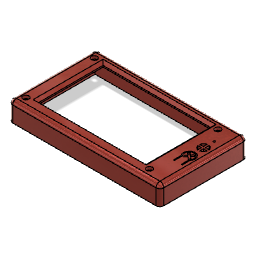
1-5i_Case_Front v4 (Autodesk Fusion 360 design; units mm, degrees)
Autodesk Fusion 360 part; units mm, degrees
sketch "Sketch1" plane through (0, 14.8501, 0) normal (0, 1, 0) x (-1, 0, 0)
  line L0 (118.407, 52.4604) -> (106.757, 52.4604)
  line L1 (106.757, 52.4604) -> (106.757, 50.3604)
  arc A0 (106.257, 49.8604) -> (106.757, 50.3604) centre (106.257, 50.3604) ccw
  line L2 (106.257, 49.8604) -> (103.757, 49.8604)
  line L3 (103.757, 49.8604) -> (103.757, 47.2604)
  arc A1 (103.257, 46.7604) -> (103.757, 47.2604) centre (103.257, 47.2604) ccw
  line L4 (103.257, 46.7604) -> (30.507, 46.7604)
  arc A2 (30.007, 47.2604) -> (30.507, 46.7604) centre (30.507, 47.2604) ccw
  line L5 (30.007, 47.2604) -> (30.007, 52.4604)
  line L6 (30.007, 52.4604) -> (-27.043, 52.4604)
  line L7 (-27.043, 52.4604) -> (-27.043, -23.3396)
  line L8 (-27.043, -23.3396) -> (118.407, -23.3396)
  line L9 (118.407, -23.3396) -> (118.407, 29.9604)
  line L10 (118.407, 29.9604) -> (116.257, 29.9604)
  arc A3 (115.757, 30.4604) -> (116.257, 29.9604) centre (116.257, 30.4604) ccw
  line L11 (115.757, 30.4604) -> (115.757, 43.4604)
  arc A4 (116.257, 43.9604) -> (115.757, 43.4604) centre (116.257, 43.4604) ccw
  line L12 (116.257, 43.9604) -> (118.407, 43.9604)
  line L13 (118.407, 43.9604) -> (118.407, 52.4604)
  circle A5 centre (115.807, 49.8604) radius 2.25
  circle A6 centre (115.807, -20.7396) radius 2.25
  circle A7 centre (-11.693, 49.8604) radius 2.25
  circle A8 centre (-11.693, -20.7396) radius 2.25
  circle A9 centre (115.807, 14.5604) radius 2.25
  circle A10 centre (115.807, -20.7396) radius 1.75
  circle A11 centre (115.807, 49.8604) radius 1.75
  circle A12 centre (-11.693, 49.8604) radius 1.75
  circle A13 centre (-11.693, -20.7396) radius 1.75
  circle A14 centre (-11.693, -20.7396) radius 3
  circle A15 centre (-11.693, 49.8604) radius 3
  circle A16 centre (115.807, 49.8604) radius 3
  circle A17 centre (115.807, -20.7396) radius 3
  dimension "d1" = 3.5
  dimension "d2" = 3.5
  dimension "d3" = 3.5
  dimension "d4" = 3.5
  dimension "d5" = 6
  dimension "d6" = 6
  dimension "d7" = 6
  dimension "d8" = 6
  constraint concentric A6 A10
  constraint concentric A5 A11
  constraint concentric A7 A12
  constraint concentric A8 A13
  constraint concentric A8 A14
  constraint concentric A7 A15
  constraint concentric A5 A16
  constraint concentric A6 A17
  measures "d1" diameter of A10
  measures "d2" diameter of A11
  measures "d3" diameter of A12
  measures "d4" diameter of A13
  measures "d5" diameter of A14
  measures "d6" diameter of A15
  measures "d7" diameter of A16
  measures "d8" diameter of A17
extrude "Extrude1" add sketch "Sketch1" along normal blind 4.3 contours L0 L13 A16 | L0 A16 | L13 A16 | L9 A17 | L8 L9 A17 | L8 A17 | L8 A14 | L8 A14 | L6 A15 | L6 A15 | A5 | A6 | A7 | A8 picked at (115.8631, 52.3416) picked at (115.751, -23.2209) makes body 1 at (-115.7322, 17.7168, 46.8613) makes body 2 at (8.7079, 17.7168, 50.1591) makes body 3 at (-116.6196, 16.2834, -23.6275) makes body 4 at (8.7079, 17.7168, -20.4409)
sketch "Sketch2" plane through (0, 19.1501, 0) normal (0, 1, 0) x (-1, 0, 0)
  circle A0 centre (115.807, -20.7396) radius 1.75
  circle A1 centre (115.807, -20.7396) radius 3
  line L0 (120.907, -26.5896) -> (-29.043, -26.5896)
  line L1 (-29.043, -26.5896) -> (-29.043, 56.4604)
  line L2 (-29.043, 56.4604) -> (120.907, 56.4604)
  line L3 (120.907, 56.4604) -> (120.907, -26.5896)
  line L4 (109.007, -23.0896) -> (-5.793, -23.0896)
  line L5 (-5.793, -23.0896) -> (-5.793, 45.4104)
  line L6 (-5.793, 45.4104) -> (109.007, 45.4104)
  line L7 (109.007, 45.4104) -> (109.007, -23.0896)
  line L8 (-27.043, -23.3396) -> (118.407, -23.3396)
  line L9 (108.757, -22.8396) -> (-5.543, -22.8396)
  line L10 (108.757, 45.1604) -> (108.757, -22.8396)
  line L11 (-5.543, 45.1604) -> (108.757, 45.1604)
  line L12 (-5.543, -22.8396) -> (-5.543, 45.1604)
  line L13 (110.507, -24.5896) -> (-8.293, -24.5896)
  line L14 (-27.043, 52.4604) -> (-27.043, -23.3396)
  circle A2 centre (115.807, 49.8604) radius 1.75
  circle A3 centre (-11.693, 49.8604) radius 1.75
  circle A4 centre (-11.693, -20.7396) radius 1.75
  circle A5 centre (-20.543, 2.9604) radius 5
  line L15 (-25.4419, 1.9604) -> (-15.644, 1.9604)
  line L16 (-15.644, 1.9604) -> (-15.644, 3.9604)
  line L17 (-15.644, 3.9604) -> (-25.4419, 3.9604)
  line L18 (-25.4419, 3.9604) -> (-25.4419, 1.9604)
  line L19 (-25.4419, 1.9604) -> (-15.644, 3.9604) construction
  line L20 (-15.644, 1.9604) -> (-25.4419, 3.9604) construction
  line L21 (-21.543, -1.9386) -> (-19.543, -1.9386)
  line L22 (-19.543, -1.9386) -> (-19.543, 7.8593)
  line L23 (-19.543, 7.8593) -> (-21.543, 7.8593)
  line L24 (-21.543, 7.8593) -> (-21.543, -1.9386)
  line L25 (-21.543, -1.9386) -> (-19.543, 7.8593) construction
  line L26 (-19.543, -1.9386) -> (-21.543, 7.8593) construction
  arc A6 (-20.4667, 7.9598) -> (-16.4773, 5.8707) centre (-20.543, 2.9604) ccw
  circle A7 centre (-20.543, 14.4604) radius 1.5
  circle A8 centre (-20.543, -8.0396) radius 1
  circle A9 centre (-20.543, -8.0396) radius 1.5
  line L27 (-17.043, 21.2811) -> (-17.043, 28.2811)
  line L28 (-24.043, 28.2811) -> (-24.043, 21.2811)
  line L29 (-16.043, 21.679) -> (-16.043, 29.2811)
  line L30 (-25.043, 29.2811) -> (-25.043, 21.679)
  arc A10 (-25.043, 21.679) -> (-16.043, 21.679) centre (-20.543, 17.7104) ccw
  line L31 (-24.043, 28.2811) -> (-24.043, 29.2811)
  line L32 (-17.043, 28.2811) -> (-17.043, 29.2811)
  arc A11 (-24.043, 21.2811) -> (-17.043, 21.2811) centre (-20.543, 17.7104) ccw
  line L33 (-16.043, 29.2811) -> (-17.043, 29.2811)
  line L34 (-24.043, 29.2811) -> (-25.043, 29.2811)
  point P0 (5.957, 55.4604)
  point P1 (-20.543, 2.9604)
  point P2 (-20.543, 2.9604)
  dimension "d12" = 0.25
  dimension "d13" = 0.25
  dimension "d14" = 0.25
  dimension "d15" = 2.5
  dimension "d16" = 2
  dimension "d17" = 1
  dimension "d18" = 2
  dimension "d21" = 10
  dimension "d22" = 2
  dimension "d23" = 2
  dimension "d24" = 10
  dimension "d26" = 3.25
  dimension "d27" = 2
  dimension "d28" = 7
  dimension "d29" = 7
  dimension "d55" = 0.25
  constraint horizontal L0
  constraint vertical L1
  constraint horizontal L2
  constraint vertical L3
  constraint horizontal L4
  constraint vertical L5
  constraint horizontal L6
  constraint vertical L7
  constraint perpendicular L15 L16
  constraint parallel L15 L17
  constraint parallel L16 L18
  constraint horizontal L15
  constraint coincident L19 P2
  constraint coincident L20 P2
  constraint coincident P2 P1
  constraint perpendicular L21 L22
  constraint parallel L21 L23
  constraint parallel L22 L24
  constraint horizontal L21
  constraint coincident L25 P2
  constraint coincident L26 P2
  constraint concentric A5 A6
  constraint coincident A5 L15.start
  constraint vertical A10.centre A7.centre
  constraint concentric A8 A9
  constraint vertical L27
  constraint vertical L28
  constraint parallel L27 L29
  constraint parallel L28 L30
  constraint coincident L31.end L33
  constraint perpendicular L31 L33
  constraint perpendicular L32 L33
  constraint collinear L33 L34
  constraint coincident A5 L21.end
  measures "d12" distance of L7 L10
  measures "d13" distance of L6 L11
  measures "d14" distance of L5 L12
  measures "d15" distance of L3 L8.end
  measures "d16" distance of L0 L13
  measures "d17" distance of L2 P0
  measures "d18" distance of L1 L14
  measures "d21" diameter of A5
  measures "d22" distance of L15 L17
  measures "d23" distance of L22.end L23.end
  measures "d24" diameter of A11
  measures "d26" distance of A7.centre A10.centre
  measures "d27" diameter of A8
  measures "d28" distance of L28.end L27.start
  measures "d29" distance of L28.end L28.start
  measures "d55" distance of L4 L9
extrude "Extrude2" add sketch "Sketch2" along normal blind 4 contours A1 L8 | A1 L8 | L0 L1 L2 L3 | A5 L16 A6 | L15 L16 L17 L22 | L15 L17 L22 L24 | L17 L22 L23 L24 | A5 L21 A6 | L15 L21 L22 L24 | A5 L23 A6 | L15 L17 L18 L24 | A5 L18 A6 | A7 | A9 bodies 1 2 3 4
sketch "Sketch3" plane through (0, 23.1501, 0) normal (0, 1, 0) x (-1, 0, 0)
  arc A0 (-19.543, -1.9386) -> (-15.644, 1.9604) centre (-20.543, 2.9604) ccw
  line L0 (-19.543, -1.9386) -> (-19.543, 1.9604)
  line L1 (-19.543, 1.9604) -> (-15.644, 1.9604)
  circle A1 centre (115.807, 49.8604) radius 1.75
  circle A2 centre (115.807, -20.7396) radius 1.75
  arc A3 (-25.4419, 1.9604) -> (-21.543, -1.9386) centre (-20.543, 2.9604) ccw
  line L2 (-25.4419, 1.9604) -> (-21.543, 1.9604)
  line L3 (-21.543, 1.9604) -> (-21.543, -1.9386)
  circle A4 centre (-11.693, -20.7396) radius 1.75
  circle A5 centre (-11.693, 49.8604) radius 1.75
  arc A6 (-21.543, 7.8593) -> (-25.4419, 3.9604) centre (-20.543, 2.9604) ccw
  line L4 (-21.543, 7.8593) -> (-21.543, 3.9604)
  line L5 (-21.543, 3.9604) -> (-25.4419, 3.9604)
  line L6 (-24.043, 29.2811) -> (-24.043, 21.2811)
  arc A7 (-24.043, 21.2811) -> (-17.043, 21.2811) centre (-20.543, 17.7104) ccw
  line L7 (-17.043, 21.2811) -> (-17.043, 29.2811)
  line L8 (-17.043, 29.2811) -> (-16.043, 29.2811)
  line L9 (-16.043, 29.2811) -> (-16.043, 21.679)
  arc A8 (-25.043, 21.679) -> (-16.043, 21.679) centre (-20.543, 17.7104) ccw
  line L10 (-25.043, 21.679) -> (-25.043, 29.2811)
  line L11 (-25.043, 29.2811) -> (-24.043, 29.2811)
  arc A9 (-15.644, 3.9604) -> (-19.543, 7.8593) centre (-20.543, 2.9604) ccw
  line L12 (-15.644, 3.9604) -> (-19.543, 3.9604)
  line L13 (-19.543, 3.9604) -> (-19.543, 7.8593)
  line L14 (109.007, -23.0896) -> (-5.793, -23.0896)
  line L15 (-5.793, -23.0896) -> (-5.793, 45.4104)
  line L16 (-5.793, 45.4104) -> (109.007, 45.4104)
  line L17 (109.007, 45.4104) -> (109.007, -23.0896)
  line L18 (120.907, 56.4604) -> (-29.043, 56.4604)
  line L19 (-29.043, 56.4604) -> (-29.043, -26.5896)
  line L20 (-29.043, -26.5896) -> (120.907, -26.5896)
  line L21 (120.907, -26.5896) -> (120.907, 56.4604)
  circle A10 centre (-11.693, 49.8604) radius 3
  circle A11 centre (-11.693, -20.7396) radius 3
  circle A12 centre (115.807, -20.7396) radius 3
  circle A13 centre (115.807, 49.8604) radius 3
  circle A14 centre (-20.543, -8.0396) radius 1
  dimension "d31" = 6
  dimension "d32" = 6
  dimension "d33" = 6
  dimension "d34" = 6
  constraint concentric A5 A10
  constraint concentric A4 A11
  constraint concentric A2 A12
  constraint concentric A1 A13
  measures "d31" diameter of A10
  measures "d32" diameter of A11
  measures "d33" diameter of A12
  measures "d34" diameter of A13
extrude "Extrude3" cut sketch "Sketch3" against normal blind 3 contours A10 | A11 | A12 | A13 bodies 1
sketch "Sketch4" plane through (0, 19.1501, 0) normal (0, -1, 0) x (1, 0, 0)
  circle A0 centre (11.693, -20.7396) radius 3
  circle A1 centre (-115.807, -20.7396) radius 3
  circle A2 centre (11.693, 49.8604) radius 3
  line L0 (29.043, 56.4604) -> (-120.907, 56.4604)
  line L1 (-120.907, 56.4604) -> (-120.907, -26.5896)
  line L2 (-120.907, -26.5896) -> (29.043, -26.5896)
  line L3 (29.043, -26.5896) -> (29.043, 56.4604)
  line L4 (5.793, -23.0896) -> (-109.007, -23.0896)
  line L5 (-109.007, -23.0896) -> (-109.007, 45.4104)
  line L6 (-109.007, 45.4104) -> (5.793, 45.4104)
  line L7 (5.793, 45.4104) -> (5.793, -23.0896)
  arc A3 (19.543, 7.8593) -> (15.644, 3.9604) centre (20.543, 2.9604) ccw
  line L8 (19.543, 7.8593) -> (19.543, 3.9604)
  line L9 (19.543, 3.9604) -> (15.644, 3.9604)
  line L10 (24.043, 21.2811) -> (24.043, 29.2811)
  line L11 (24.043, 29.2811) -> (25.043, 29.2811)
  line L12 (25.043, 29.2811) -> (25.043, 21.679)
  arc A4 (16.043, 21.679) -> (25.043, 21.679) centre (20.543, 17.7104) ccw
  line L13 (16.043, 21.679) -> (16.043, 29.2811)
  line L14 (16.043, 29.2811) -> (17.043, 29.2811)
  line L15 (17.043, 29.2811) -> (17.043, 21.2811)
  arc A5 (17.043, 21.2811) -> (24.043, 21.2811) centre (20.543, 17.7104) ccw
  arc A6 (25.4419, 3.9604) -> (21.543, 7.8593) centre (20.543, 2.9604) ccw
  line L16 (25.4419, 3.9604) -> (21.543, 3.9604)
  line L17 (21.543, 3.9604) -> (21.543, 7.8593)
  arc A7 (21.543, -1.9386) -> (25.4419, 1.9604) centre (20.543, 2.9604) ccw
  line L18 (21.543, -1.9386) -> (21.543, 1.9604)
  line L19 (21.543, 1.9604) -> (25.4419, 1.9604)
  arc A8 (15.644, 1.9604) -> (19.543, -1.9386) centre (20.543, 2.9604) ccw
  line L20 (15.644, 1.9604) -> (19.543, 1.9604)
  line L21 (19.543, 1.9604) -> (19.543, -1.9386)
  circle A9 centre (-115.807, 49.8604) radius 3
  circle A10 centre (20.543, 14.4604) radius 1.25
  circle A11 centre (20.543, 14.4604) radius 1.5
  circle A12 centre (20.543, -8.0396) radius 1
  dimension "d37" = 2.5
  constraint concentric A10 A11
  measures "d37" diameter of A10
extrude "Extrude4" add sketch "Sketch4" along normal blind 1.25 contours A10 bodies 1
sketch "Sketch5" plane through (0, 23.1501, 0) normal (0, 1, 0) x (-1, 0, 0)
  circle A0 centre (115.807, 49.8604) radius 3
  circle A1 centre (-11.693, 49.8604) radius 3
  circle A2 centre (115.807, -20.7396) radius 3
  circle A3 centre (-11.693, -20.7396) radius 3
  arc A4 (-19.543, -1.9386) -> (-15.644, 1.9604) centre (-20.543, 2.9604) ccw
  line L0 (-19.543, -1.9386) -> (-19.543, 1.9604)
  line L1 (-19.543, 1.9604) -> (-15.644, 1.9604)
  arc A5 (-25.4419, 1.9604) -> (-21.543, -1.9386) centre (-20.543, 2.9604) ccw
  line L2 (-25.4419, 1.9604) -> (-21.543, 1.9604)
  line L3 (-21.543, 1.9604) -> (-21.543, -1.9386)
  arc A6 (-21.543, 7.8593) -> (-25.4419, 3.9604) centre (-20.543, 2.9604) ccw
  line L4 (-21.543, 7.8593) -> (-21.543, 3.9604)
  line L5 (-21.543, 3.9604) -> (-25.4419, 3.9604)
  line L6 (-24.043, 29.2811) -> (-24.043, 21.2811)
  arc A7 (-24.043, 21.2811) -> (-17.043, 21.2811) centre (-20.543, 17.7104) ccw
  line L7 (-17.043, 21.2811) -> (-17.043, 29.2811)
  line L8 (-17.043, 29.2811) -> (-16.043, 29.2811)
  line L9 (-16.043, 29.2811) -> (-16.043, 21.679)
  arc A8 (-25.043, 21.679) -> (-16.043, 21.679) centre (-20.543, 17.7104) ccw
  line L10 (-25.043, 21.679) -> (-25.043, 29.2811)
  line L11 (-25.043, 29.2811) -> (-24.043, 29.2811)
  arc A9 (-15.644, 3.9604) -> (-19.543, 7.8593) centre (-20.543, 2.9604) ccw
  line L12 (-15.644, 3.9604) -> (-19.543, 3.9604)
  line L13 (-19.543, 3.9604) -> (-19.543, 7.8593)
  line L14 (109.007, -23.0896) -> (-5.793, -23.0896)
  line L15 (-5.793, -23.0896) -> (-5.793, 45.4104)
  line L16 (-5.793, 45.4104) -> (109.007, 45.4104)
  line L17 (109.007, 45.4104) -> (109.007, -23.0896)
  line L18 (120.907, 56.4604) -> (-29.043, 56.4604)
  line L19 (-29.043, 56.4604) -> (-29.043, -26.5896)
  line L20 (-29.043, -26.5896) -> (120.907, -26.5896)
  line L21 (120.907, -26.5896) -> (120.907, 56.4604)
  line L22 (-18.1376, 14.3615) -> (-24.2412, 19.5333)
  line L23 (-24.2412, 19.5333) -> (-22.9483, 21.0592)
  line L24 (-22.9483, 21.0592) -> (-16.8447, 15.8874)
  line L25 (-16.8447, 15.8874) -> (-18.1376, 14.3615)
  line L26 (-17.1942, 20.1157) -> (-22.3659, 14.0121)
  line L27 (-22.3659, 14.0121) -> (-23.8918, 15.305)
  line L28 (-23.8918, 15.305) -> (-18.72, 21.4086)
  line L29 (-18.72, 21.4086) -> (-17.1942, 20.1157)
  line L30 (-23.1288, 14.6586) -> (-17.9571, 20.7621) construction
  line L31 (-17.4912, 15.1245) -> (-23.5947, 20.2962) construction
  circle A10 centre (-20.543, -8.0396) radius 1
  dimension "d40" = 2
  dimension "d41" = 2
  dimension "d42" = 8
  dimension "d43" = 8
  constraint perpendicular L22 L23
  constraint parallel L22 L24
  constraint parallel L23 L25
  constraint perpendicular L26 L27
  constraint parallel L26 L28
  constraint parallel L27 L29
  constraint perpendicular L22 L26
  constraint midpoint L27 L30.start
  constraint midpoint L29 L30.end
  constraint midpoint L25 L31.start
  constraint midpoint L23 L31.end
  constraint midpoint L30 L31
  constraint midpoint A7.centre L30
  measures "d40" distance of L22.start L24.end
  measures "d41" distance of L26.end L27.end
  measures "d42" distance of L22.start L22.end
  measures "d43" distance of L26.start L26.end
extrude "Extrude5" cut sketch "Sketch5" against normal blind 1.5 contours L22 L24 L25 L26 | L22 L26 L27 L28 | L22 L24 L26 L28 | L22 L23 L24 L28 | L24 L26 L28 L29 bodies 1
sketch "Sketch6" plane through (0, 23.1501, 0) normal (0, 1, 0) x (-1, 0, 0)
  line L0 (-22.9483, 21.0592) -> (-20.6594, 19.1198)
  line L1 (-20.6594, 19.1198) -> (-18.72, 21.4086)
  line L2 (-18.72, 21.4086) -> (-17.1942, 20.1157)
  line L3 (-17.1942, 20.1157) -> (-19.1336, 17.8268)
  line L4 (-19.1336, 17.8268) -> (-16.8447, 15.8874)
  line L5 (-16.8447, 15.8874) -> (-18.1376, 14.3615)
  line L6 (-18.1376, 14.3615) -> (-20.4265, 16.3009)
  line L7 (-20.4265, 16.3009) -> (-22.3659, 14.0121)
  line L8 (-22.3659, 14.0121) -> (-23.8918, 15.305)
  line L9 (-23.8918, 15.305) -> (-21.9524, 17.5939)
  line L10 (-21.9524, 17.5939) -> (-24.2412, 19.5333)
  line L11 (-24.2412, 19.5333) -> (-22.9483, 21.0592)
  circle A0 centre (115.807, 49.8604) radius 3
  circle A1 centre (-11.693, 49.8604) radius 3
  circle A2 centre (115.807, -20.7396) radius 3
  circle A3 centre (-11.693, -20.7396) radius 3
  line L12 (109.007, -23.0896) -> (-5.793, -23.0896)
  line L13 (-5.793, -23.0896) -> (-5.793, 45.4104)
  line L14 (-5.793, 45.4104) -> (109.007, 45.4104)
  line L15 (109.007, 45.4104) -> (109.007, -23.0896)
  line L16 (-24.043, 29.2811) -> (-24.043, 21.2811)
  arc A4 (-24.043, 21.2811) -> (-17.043, 21.2811) centre (-20.543, 17.7104) ccw
  line L17 (-17.043, 21.2811) -> (-17.043, 29.2811)
  line L18 (-17.043, 29.2811) -> (-16.043, 29.2811)
  line L19 (-16.043, 29.2811) -> (-16.043, 21.679)
  arc A5 (-25.043, 21.679) -> (-16.043, 21.679) centre (-20.543, 17.7104) ccw
  line L20 (-25.043, 21.679) -> (-25.043, 29.2811)
  line L21 (-25.043, 29.2811) -> (-24.043, 29.2811)
  arc A6 (-19.543, -1.9386) -> (-15.644, 1.9604) centre (-20.543, 2.9604) ccw
  line L22 (-19.543, -1.9386) -> (-19.543, 1.9604)
  line L23 (-19.543, 1.9604) -> (-15.644, 1.9604)
  arc A7 (-25.4419, 1.9604) -> (-21.543, -1.9386) centre (-20.543, 2.9604) ccw
  line L24 (-25.4419, 1.9604) -> (-21.543, 1.9604)
  line L25 (-21.543, 1.9604) -> (-21.543, -1.9386)
  arc A8 (-15.644, 3.9604) -> (-19.543, 7.8593) centre (-20.543, 2.9604) ccw
  line L26 (-15.644, 3.9604) -> (-19.543, 3.9604)
  line L27 (-19.543, 3.9604) -> (-19.543, 7.8593)
  circle A9 centre (-20.543, -8.0396) radius 1
  arc A10 (-21.543, 7.8593) -> (-25.4419, 3.9604) centre (-20.543, 2.9604) ccw
  line L28 (-21.543, 7.8593) -> (-21.543, 3.9604)
  line L29 (-21.543, 3.9604) -> (-25.4419, 3.9604)
  line L30 (120.907, 56.4604) -> (-29.043, 56.4604)
  line L31 (-29.043, 56.4604) -> (-29.043, -26.5896)
  line L32 (-29.043, -26.5896) -> (120.907, -26.5896)
  line L33 (120.907, -26.5896) -> (120.907, 56.4604)
  line L34 (120.907, -26.5896) -> (123.907, -26.5896)
  line L35 (123.907, -26.5896) -> (123.907, 56.4604)
  line L36 (123.907, 56.4604) -> (120.907, 56.4604)
  line L37 (120.907, 56.4604) -> (120.907, -26.5896)
  line L38 (-29.043, -26.5896) -> (-32.043, -26.5896)
  line L39 (-32.043, -26.5896) -> (-32.043, 56.4604)
  line L40 (-32.043, 56.4604) -> (-29.043, 56.4604)
  line L41 (-29.043, 56.4604) -> (-29.043, -26.5896)
  line L42 (-32.043, 56.4604) -> (123.907, 56.4604)
  line L43 (123.907, 56.4604) -> (123.907, 59.4604)
  line L44 (123.907, 59.4604) -> (-32.043, 59.4604)
  line L45 (-32.043, 59.4604) -> (-32.043, 56.4604)
  line L46 (123.907, -26.5896) -> (-32.043, -26.5896)
  line L47 (-32.043, -26.5896) -> (-32.043, -30.5896)
  line L48 (-32.043, -30.5896) -> (123.907, -30.5896)
  line L49 (123.907, -30.5896) -> (123.907, -26.5896)
  dimension "d46" = 3
  dimension "d47" = 4
  dimension "d48" = 3
  dimension "d49" = 3
  constraint horizontal L34
  constraint vertical L35
  constraint horizontal L36
  constraint vertical L37
  constraint coincident L32.end L33.start
  constraint horizontal L38
  constraint vertical L39
  constraint horizontal L40
  constraint vertical L41
  constraint coincident L31.end L32.start
  constraint horizontal L42
  constraint vertical L43
  constraint horizontal L44
  constraint vertical L45
  constraint horizontal L46
  constraint vertical L47
  constraint horizontal L48
  constraint vertical L49
  constraint coincident L35.end L36.start
  constraint coincident L30.start L42
  constraint coincident L38.end L39.start
  measures "d46" distance of L35.end L43.end
  measures "d47" distance of L34.end L48.end
  measures "d48" distance of L35 L37
  measures "d49" distance of L39 L41
extrude "Extrude6" add sketch "Sketch6" against normal blind 20 contours L33 L34 L35 L36 L37 L42 L46 | L30 L36 L40 L42 L43 L44 L45 | L31 L38 L39 L40 L41 L42 L46 | L32 L34 L38 L46 L47 L48 L49 bodies 1
chamfer "Chamfer1" distance 2.5 angle 50 4 edges at (-51.607, 23.1501, -23.0896) (-109.007, 23.1501, 11.1604) (-51.607, 23.1501, 45.4104) (5.793, 23.1501, 11.1604) measured on face at (23.8819, 23.1501, 45.9058) measured on face at (23.8819, 23.1501, 45.9058) measured on face at (23.8819, 23.1501, 45.9058) measured on face at (23.8819, 23.1501, 45.9058) on bodies 1
chamfer "Chamfer2" distance 4 angle 45 8 edges at (-45.932, 23.1501, -30.5896) (-123.907, 23.1501, 14.4354) (-123.907, 13.1501, -30.5896) (-123.907, 13.1501, 59.4604) (-45.932, 23.1501, 59.4604) (32.043, 23.1501, 14.4354) (32.043, 13.1501, 59.4604) (32.043, 13.1501, -30.5896) on bodies 1
sketch "Sketch7" plane through (-120.907, 0, 0) normal (1, 0, 0) x (0, 0, -1)
  line L0 (-56.4604, 3.1501) -> (26.5896, 3.1501)
  line L1 (26.5896, 3.1501) -> (26.5896, 19.1501)
  line L2 (26.5896, 19.1501) -> (-56.4604, 19.1501)
  line L3 (-56.4604, 19.1501) -> (-56.4604, 3.1501)
  line L4 (-26.6604, 17.1501) -> (-45.1604, 17.1501)
  line L5 (-45.1604, 17.1501) -> (-45.1604, 7.4001)
  line L6 (-45.1604, 7.4001) -> (-26.6604, 7.4001)
  line L7 (-26.6604, 7.4001) -> (-26.6604, 17.1501)
  point P0 (-28.6604, 11.4001)
  point P1 (-43.1604, 11.4001)
  point P2 (-28.6604, 11.4001)
  dimension "d56" = 2
  dimension "d57" = 2
  dimension "d58" = 2
  dimension "d59" = 4
  constraint horizontal L4
  constraint vertical L5
  constraint horizontal L6
  constraint vertical L7
  measures "d56" distance of L7 P2
  measures "d57" distance of L5 P1
  measures "d58" distance of L2 L4
  measures "d59" distance of L6 P2
extrude "Extrude7" cut sketch "Sketch7" against normal blind 20 contours L4 L5 L6 L7 bodies 1
chamfer "Chamfer3" distance 1.5 angle 45 4 edges at (-123.907, 12.2751, 45.1604) (-123.907, 12.2751, 26.6604) (-123.907, 17.1501, 35.9104) (-123.907, 7.4001, 35.9104) on bodies 1
delete_face "DeleteFace1" 4 faces at (29.3763, 20.4834, -27.923) (29.3763, 20.4834, 56.7937) (-121.2404, 20.4834, 56.7937) (-121.2404, 20.4834, -27.923) on bodies 1
delete_face "DeleteFace2" 4 faces at (-122.5737, 20.4834, 28.1104) (-21.2737, 20.4834, -29.2563) (-21.2737, 20.4834, 58.127) (29.3763, 21.8168, 28.1104) on bodies 1
delete_face "DeleteFace3" 4 faces at (30.7096, 9.8168, 56.7937) (30.7096, 16.4834, -27.923) (-122.5737, 9.8168, -27.923) (-122.5737, 9.8168, 56.7937) on bodies 1
fillet "Fillet1" radius 4 8 edges at (-123.907, 23.1501, 14.4354) (-123.907, 13.1501, -30.5896) (-45.932, 23.1501, -30.5896) (-45.932, 23.1501, 59.4604) (-123.907, 13.1501, 59.4604) (32.043, 13.1501, 59.4604) (32.043, 23.1501, 14.4354) (32.043, 13.1501, -30.5896) on bodies 1
delete_face "DeleteFace4" 1 faces at (-123.407, 13.9001, 25.6604) on bodies 1
delete_face "DeleteFace5" 1 faces at (-123.407, 18.1501, 39.4937) on bodies 1
delete_face "DeleteFace6" 1 faces at (-123.407, 6.4001, 39.4937) on bodies 1
delete_face "DeleteFace7" 1 faces at (-122.907, 10.6501, 45.6604) on bodies 1
delete_face "DeleteFace8" 1 faces at (-122.907, 13.9001, 45.1604) on bodies 1
delete_face "DeleteFace9" 1 faces at (7.4596, 22.157, 22.577) on bodies 1
extrude "Extrude8" add 1 faces at (5.793, 22.157, 22.577) along direction (-1, 0, 0) blind 2.25 on bodies 1 bodies 1
delete_face "DeleteFace10" 1 faces at (-72.3237, 22.157, -24.7563) on bodies 1
extrude "Extrude9" add 1 faces at (-33.9737, 20.8237, -23.0896) along direction (0, 0, 1) blind 2 on bodies 1 bodies 1
delete_face "DeleteFace11" 1 faces at (-110.6737, 22.157, 24.077) on bodies 1
extrude "Extrude10" add 1 faces at (-109.007, 20.8237, 1.077) along direction (1, 0, 0) blind 1.75 on bodies 1 bodies 1
chamfer "Chamfer4" distance 2.5 angle 50 3 edges at (-107.257, 23.1501, 13.4104) (-51.857, 23.1501, -21.0896) (3.543, 23.1501, 13.4104) measured on face at (-107.257, 20.8237, 1.077) measured on face at (-70.3237, 20.4834, -21.0896) measured on face at (3.543, 20.8237, 1.077) on bodies 1
